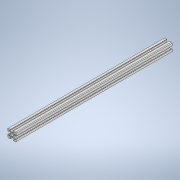
# Autodesk Inventor part: aluminum profile
Saved by Autodesk Inventor 2022 (Build 260153000, 153)
## iProperties
Created: 2021-10-04
Part Number: aluminum profile
Material: Generic
Document SubType Name: Modeling
Designer: tecware
Density: 1 g/cm^3
Appearance: Default
Author: tecware
Autodesk Inventor part; units mm, degrees
ref_plane "YZ Plane" through (0, 0, 0) normal (1, 0, 0) x (0, 1, 0)
ref_plane "XZ Plane" through (0, 0, 0) normal (0, 1, 0) x (-1, 0, 0)
ref_plane "XY Plane" through (0, 0, 0) normal (0, 0, 1) x (1, 0, 0)
sketch "Sketch1" plane through (0, 0, 0) normal (0, 0, 1) x (1, 0, 0)
  line L0 (21.2061, 16.2389) -> (17.5361, 16.2389) projected
  arc A0 (17.5361, 16.2389) -> (16.0361, 14.7389) centre (17.5361, 14.7389) ccw projected
  line L1 (16.0361, 14.7389) -> (16.0361, 11.0689) projected
  arc A1 (17.6093, 9.3921) -> (18.0361, 9.5689) centre (17.7861, 9.5689) ccw projected
  line L2 (18.0361, 9.5689) -> (18.0361, 11.3389) projected
  arc A2 (22.0361, 8.1377) -> (21.4503, 9.5519) centre (20.0361, 8.1377) ccw projected
  line L3 (22.0361, 8.1377) -> (22.0361, 6.5766) projected
  arc A3 (22.0361, 6.5766) -> (22.0909, 6.4204) centre (22.2861, 6.5766) ccw projected
  line L4 (22.0909, 6.4204) -> (22.2361, 6.2389) projected
  line L5 (22.2361, 6.2389) -> (22.0909, 6.0574) projected
  arc A4 (22.0909, 6.0574) -> (22.0361, 5.9012) centre (22.2861, 5.9012) ccw projected
  line L6 (22.0361, 5.9012) -> (22.0361, 4.3401) projected
  arc A5 (21.4503, 2.9259) -> (22.0361, 4.3401) centre (20.0361, 4.3401) ccw projected
  line L7 (21.4503, 2.9259) -> (19.7562, 1.2318) projected
  arc A6 (19.0491, 0.9389) -> (19.7562, 1.2318) centre (19.0491, 1.9389) ccw projected
  line L8 (19.0491, 0.9389) -> (18.2361, 0.9389) projected
  arc A7 (18.0361, 1.1389) -> (18.2361, 0.9389) centre (18.2361, 1.1389) ccw projected
  line L9 (18.0361, 1.1389) -> (18.0361, 2.9089) projected
  arc A8 (18.0361, 2.9089) -> (17.6093, 3.0857) centre (17.7861, 2.9089) ccw projected
  line L10 (17.6093, 3.0857) -> (16.1093, 1.5857) projected
  arc A9 (16.1093, 1.5857) -> (16.0361, 1.4089) centre (16.2861, 1.4089) ccw projected
  line L11 (16.0361, 1.4089) -> (16.0361, -2.2611) projected
  arc A10 (16.0361, -2.2611) -> (17.5361, -3.7611) centre (17.5361, -2.2611) ccw projected
  line L12 (17.5361, -3.7611) -> (21.2061, -3.7611) projected
  arc A11 (21.2061, -3.7611) -> (21.3829, -3.6879) centre (21.2061, -3.5111) ccw projected
  line L13 (21.3829, -3.6879) -> (22.8829, -2.1879) projected
  arc A12 (22.8829, -2.1879) -> (22.7061, -1.7611) centre (22.7061, -2.0111) ccw projected
  line L14 (22.7061, -1.7611) -> (20.9361, -1.7611) projected
  arc A13 (20.7361, -1.5611) -> (20.9361, -1.7611) centre (20.9361, -1.5611) ccw projected
  line L15 (20.7361, -1.5611) -> (20.7361, -0.7481) projected
  arc A14 (21.029, -0.041) -> (20.7361, -0.7481) centre (21.7361, -0.7481) ccw projected
  line L16 (21.029, -0.041) -> (22.7231, 1.6531) projected
  arc A15 (24.1373, 2.2389) -> (22.7231, 1.6531) centre (24.1373, 0.2389) ccw projected
  line L17 (24.1373, 2.2389) -> (25.6984, 2.2389) projected
  arc A16 (25.6984, 2.2389) -> (25.8546, 2.2937) centre (25.6984, 2.4889) ccw projected
  line L18 (25.8546, 2.2937) -> (26.0361, 2.4389) projected
  line L19 (26.0361, 2.4389) -> (26.2176, 2.2937) projected
  arc A17 (26.2176, 2.2937) -> (26.3738, 2.2389) centre (26.3738, 2.4889) ccw projected
  line L20 (26.3738, 2.2389) -> (27.9349, 2.2389) projected
  arc A18 (29.3491, 1.6531) -> (27.9349, 2.2389) centre (27.9349, 0.2389) ccw projected
  line L21 (29.3491, 1.6531) -> (31.0432, -0.041) projected
  arc A19 (31.3361, -0.7481) -> (31.0432, -0.041) centre (30.3361, -0.7481) ccw projected
  line L22 (31.3361, -0.7481) -> (31.3361, -1.5611) projected
  arc A20 (31.1361, -1.7611) -> (31.3361, -1.5611) centre (31.1361, -1.5611) ccw projected
  line L23 (31.1361, -1.7611) -> (29.3661, -1.7611) projected
  arc A21 (29.3661, -1.7611) -> (29.1893, -2.1879) centre (29.3661, -2.0111) ccw projected
  line L24 (29.1893, -2.1879) -> (30.6893, -3.6879) projected
  arc A22 (30.6893, -3.6879) -> (30.8661, -3.7611) centre (30.8661, -3.5111) ccw projected
  line L25 (30.8661, -3.7611) -> (34.5361, -3.7611) projected
  arc A23 (34.5361, -3.7611) -> (36.0361, -2.2611) centre (34.5361, -2.2611) ccw projected
  line L26 (36.0361, -2.2611) -> (36.0361, 1.4089) projected
  arc A24 (36.0361, 1.4089) -> (35.9629, 1.5857) centre (35.7861, 1.4089) ccw projected
  line L27 (35.9629, 1.5857) -> (34.4629, 3.0857) projected
  arc A25 (34.4629, 3.0857) -> (34.0361, 2.9089) centre (34.2861, 2.9089) ccw projected
  line L28 (34.0361, 2.9089) -> (34.0361, 1.1389) projected
  arc A26 (33.8361, 0.9389) -> (34.0361, 1.1389) centre (33.8361, 1.1389) ccw projected
  line L29 (33.8361, 0.9389) -> (33.0231, 0.9389) projected
  arc A27 (32.316, 1.2318) -> (33.0231, 0.9389) centre (33.0231, 1.9389) ccw projected
  line L30 (32.316, 1.2318) -> (30.6219, 2.9259) projected
  arc A28 (30.0361, 4.3401) -> (30.6219, 2.9259) centre (32.0361, 4.3401) ccw projected
  line L31 (30.0361, 4.3401) -> (30.0361, 5.9012) projected
  arc A29 (30.0361, 5.9012) -> (29.9813, 6.0574) centre (29.7861, 5.9012) ccw projected
  line L32 (29.9813, 6.0574) -> (29.8361, 6.2389) projected
  line L33 (29.8361, 6.2389) -> (29.9813, 6.4204) projected
  arc A30 (29.9813, 6.4204) -> (30.0361, 6.5766) centre (29.7861, 6.5766) ccw projected
  line L34 (30.0361, 6.5766) -> (30.0361, 8.1377) projected
  arc A31 (30.6219, 9.5519) -> (30.0361, 8.1377) centre (32.0361, 8.1377) ccw projected
  line L35 (30.6219, 9.5519) -> (32.316, 11.246) projected
  arc A32 (33.0231, 11.5389) -> (32.316, 11.246) centre (33.0231, 10.5389) ccw projected
  line L36 (33.0231, 11.5389) -> (33.8361, 11.5389) projected
  arc A33 (34.0361, 11.3389) -> (33.8361, 11.5389) centre (33.8361, 11.3389) ccw projected
  line L37 (34.0361, 11.3389) -> (34.0361, 9.5689) projected
  arc A34 (34.0361, 9.5689) -> (34.4629, 9.3921) centre (34.2861, 9.5689) ccw projected
  line L38 (34.4629, 9.3921) -> (35.9629, 10.8921) projected
  arc A35 (35.9629, 10.8921) -> (36.0361, 11.0689) centre (35.7861, 11.0689) ccw projected
  line L39 (36.0361, 11.0689) -> (36.0361, 14.7389) projected
  arc A36 (36.0361, 14.7389) -> (34.5361, 16.2389) centre (34.5361, 14.7389) ccw projected
  line L40 (34.5361, 16.2389) -> (30.8661, 16.2389) projected
  arc A37 (30.8661, 16.2389) -> (30.6893, 16.1657) centre (30.8661, 15.9889) ccw projected
  line L41 (30.6893, 16.1657) -> (29.1893, 14.6657) projected
  arc A38 (29.1893, 14.6657) -> (29.3661, 14.2389) centre (29.3661, 14.4889) ccw projected
  line L42 (29.3661, 14.2389) -> (31.1361, 14.2389) projected
  arc A39 (31.3361, 14.0389) -> (31.1361, 14.2389) centre (31.1361, 14.0389) ccw projected
  line L43 (31.3361, 14.0389) -> (31.3361, 13.2259) projected
  arc A40 (31.0432, 12.5188) -> (31.3361, 13.2259) centre (30.3361, 13.2259) ccw projected
  line L44 (31.0432, 12.5188) -> (29.3491, 10.8247) projected
  arc A41 (27.9349, 10.2389) -> (29.3491, 10.8247) centre (27.9349, 12.2389) ccw projected
  line L45 (27.9349, 10.2389) -> (26.3738, 10.2389) projected
  arc A42 (26.3738, 10.2389) -> (26.2176, 10.1841) centre (26.3738, 9.9889) ccw projected
  line L46 (26.2176, 10.1841) -> (26.0361, 10.0389) projected
  line L47 (26.0361, 10.0389) -> (25.8546, 10.1841) projected
  arc A43 (25.8546, 10.1841) -> (25.6984, 10.2389) centre (25.6984, 9.9889) ccw projected
  line L48 (25.6984, 10.2389) -> (24.1373, 10.2389) projected
  arc A44 (22.7231, 10.8247) -> (24.1373, 10.2389) centre (24.1373, 12.2389) ccw projected
  line L49 (22.7231, 10.8247) -> (21.029, 12.5188) projected
  arc A45 (20.7361, 13.2259) -> (21.029, 12.5188) centre (21.7361, 13.2259) ccw projected
  line L50 (20.7361, 13.2259) -> (20.7361, 14.0389) projected
  arc A46 (20.9361, 14.2389) -> (20.7361, 14.0389) centre (20.9361, 14.0389) ccw projected
  line L51 (20.9361, 14.2389) -> (22.7061, 14.2389) projected
  arc A47 (22.7061, 14.2389) -> (22.8829, 14.6657) centre (22.7061, 14.4889) ccw projected
  arc A48 (21.3829, 16.1657) -> (21.2061, 16.2389) centre (21.2061, 15.9889) ccw projected
  line L52 (21.2061, 16.2389) -> (17.5361, 16.2389) projected
  arc A49 (17.5361, 16.2389) -> (16.0361, 14.7389) centre (17.5361, 14.7389) ccw projected
  line L53 (16.0361, 14.7389) -> (16.0361, 11.0689) projected
  arc A50 (16.0361, 11.0689) -> (16.1093, 10.8921) centre (16.2861, 11.0689) ccw projected
  line L54 (16.1093, 10.8921) -> (17.6093, 9.3921) projected
  arc A51 (17.6093, 9.3921) -> (18.0361, 9.5689) centre (17.7861, 9.5689) ccw projected
  line L55 (18.0361, 9.5689) -> (18.0361, 11.3389) projected
  arc A52 (18.2361, 11.5389) -> (18.0361, 11.3389) centre (18.2361, 11.3389) ccw projected
  line L56 (18.2361, 11.5389) -> (19.0491, 11.5389) projected
  arc A53 (19.7562, 11.246) -> (19.0491, 11.5389) centre (19.0491, 10.5389) ccw projected
  line L57 (19.7562, 11.246) -> (21.4503, 9.5519) projected
  circle A54 centre (26.0361, 6.2389) radius 2.5 projected
  line L58 (17.7861, 9.3189) -> (16.2861, 9.3189)
  line L59 (16.0361, 9.5689) -> (16.0361, 11.0689)
  arc A55 (16.0361, 9.5689) -> (16.2861, 9.3189) centre (16.2861, 9.5689) ccw
  line L60 (19, 6.2389) -> (36.0361, 6.2389) construction
  line L61 (26.0361, 14.1377) -> (26.0361, -0.041) construction
  line L62 (17.7861, 3.1589) -> (16.2861, 3.1589)
  line L63 (16.0361, 2.9089) -> (16.0361, 1.4089)
  arc A56 (16.2861, 3.1589) -> (16.0361, 2.9089) centre (16.2861, 2.9089) ccw
  line L64 (34.2861, 9.3189) -> (35.7861, 9.3189)
  line L65 (36.0361, 9.5689) -> (36.0361, 11.0689)
  arc A57 (35.7861, 9.3189) -> (36.0361, 9.5689) centre (35.7861, 9.5689) ccw
  line L66 (36.0361, 2.9089) -> (36.0361, 1.4089)
  line L67 (34.2861, 3.1589) -> (35.7861, 3.1589)
  arc A58 (36.0361, 2.9089) -> (35.7861, 3.1589) centre (35.7861, 2.9089) ccw
  line L68 (17.5361, 14.7389) -> (26.0361, 6.2389)
  line L69 (22.9561, 14.4889) -> (22.9561, 15.9889)
  line L70 (22.7061, 16.2389) -> (21.2061, 16.2389)
  arc A59 (22.9561, 15.9889) -> (22.7061, 16.2389) centre (22.7061, 15.9889) ccw
  line L71 (29.3661, 16.2389) -> (30.8661, 16.2389)
  arc A60 (29.3661, 16.2389) -> (29.1161, 15.9889) centre (29.3661, 15.9889) ccw
  line L72 (29.1161, 14.4889) -> (29.1161, 15.9889)
  line L73 (22.7061, -3.7611) -> (21.2061, -3.7611)
  arc A61 (22.7061, -3.7611) -> (22.9561, -3.5111) centre (22.7061, -3.5111) ccw
  line L74 (22.9561, -2.0111) -> (22.9561, -3.5111)
  line L75 (29.1161, -2.0111) -> (29.1161, -3.5111)
  line L76 (29.3661, -3.7611) -> (30.8661, -3.7611)
  arc A62 (29.1161, -3.5111) -> (29.3661, -3.7611) centre (29.3661, -3.5111) ccw
  point P0 (0, 0)
  constraints: 38 end point, 28 symmetric about line, 17 point on circle, 8 centre point, 1 horizontal, 1 perpendicular, 1 tangent, 1 vertical, 7 other
extrude "Extrusion1" add sketch "Sketch1" along normal blind 370
body "Solid1"
